Nema 8 901 (Autodesk Fusion 360 design; units mm, degrees)
Autodesk Fusion 360 part; units mm, degrees
sketch "Sketch1" plane through (0, 0, 0) normal (0, 0, 1) x (1, 0, 0)
  line L0 (10.15, -10.15) -> (-10.15, -10.15)
  line L1 (-10.15, -10.15) -> (-10.15, 10.15)
  line L2 (-10.15, 10.15) -> (10.15, 10.15)
  line L3 (10.15, 10.15) -> (10.15, -10.15)
  line L4 (10.15, -10.15) -> (-10.15, 10.15) construction
  line L5 (-10.15, -10.15) -> (10.15, 10.15) construction
  dimension "d1" = 20.3
  dimension "d2" = 20.3
  constraint perpendicular L0 L1
  constraint parallel L0 L2
  constraint parallel L1 L3
  constraint horizontal L0
  constraint coincident L4 origin
  constraint coincident L5 origin
  measures "d1" distance of L1.end L2.end
  measures "d2" distance of L0.end L1.end
extrude "Extrude1" add sketch "Sketch1" along normal blind 28
sketch "Sketch2" plane through (0, 0, 28) normal (0, 0, 1) x (-1, 0, 0)
  line L0 (-10.15, -10.15) -> (10.15, -10.15)
  line L1 (10.15, -10.15) -> (10.15, 10.15)
  line L2 (10.15, 10.15) -> (-10.15, 10.15)
  line L3 (-10.15, 10.15) -> (-10.15, -10.15)
  line L4 (-11, 11) -> (11, 11)
  line L5 (11, 11) -> (11, -11)
  line L6 (11, -11) -> (-11, -11)
  line L7 (-11, -11) -> (-11, 11)
  line L8 (-11, 11) -> (11, -11) construction
  line L9 (11, 11) -> (-11, -11) construction
  dimension "d5" = 22
  dimension "d6" = 22
  constraint perpendicular L4 L5
  constraint parallel L4 L6
  constraint parallel L5 L7
  constraint horizontal L4
  constraint coincident L8 origin
  constraint coincident L9 origin
  measures "d5" distance of L4.end L5.end
  measures "d6" distance of L5.end L6.end
extrude "Extrude2" add sketch "Sketch2" along normal blind 3 contours L0 L1 L2 L3 | L4 L5 L6 L7
sketch "Sketch3" plane through (0, 0, 31) normal (0, 0, 1) x (-1, 0, 0)
  line L0 (-11, -11) -> (11, -11)
  line L1 (11, -11) -> (11, 11)
  line L2 (11, 11) -> (-11, 11)
  line L3 (-11, 11) -> (-11, -11)
  circle A0 centre (0, 0) radius 11
  dimension "d9" = 22
  constraint coincident A0.centre origin
  measures "d9" diameter of A0
extrude "Extrude3" add sketch "Sketch3" along normal blind 24.95 contours A0
fillet "Fillet1" radius 0.5 1 faces at (0, 11, 47.6333)
sketch "Sketch4" plane through (0, 0, 55.95) normal (0, 0, 1) x (-1, 0, 0)
  circle A0 centre (0, 0) radius 11
  circle A1 centre (0, 0) radius 10.5
  constraint coincident A0.centre A1.centre
extrude "Extrude4" add sketch "Sketch4" along normal blind 3 contours A0 | A1
fillet "Fillet2" radius 0.5 1 faces at (-10.9863, 0.5483, 57.95)
fillet "Fillet3" radius 2 4 edges at (-10.15, -10.15, 14) (10.15, -10.15, 14) (10.15, 10.15, 14) (-10.15, 10.15, 14)
sketch "Sketch5" plane through (0, 0, 58.95) normal (0, 0, 1) x (-1, 0, 0)
  circle A0 centre (0, 0) radius 10.5
  circle A1 centre (0, 0) radius 6.5
  dimension "d17" = 13
  constraint coincident A0.centre A1.centre
  measures "d17" diameter of A1
extrude "Extrude5" add sketch "Sketch5" along normal blind 2 contours A1
fillet "Fillet4" radius 0.5 1 edges at (6.0601, 2.3505, 60.95)
sketch "Sketch6" plane through (0, 0, 60.95) normal (0, 0, 1) x (-1, 0, 0)
  circle A0 centre (0, 0) radius 6
  circle A1 centre (0, 0) radius 3
  dimension "d21" = 6
  constraint coincident A0.centre A1.centre
  measures "d21" diameter of A1
extrude "Extrude6" add sketch "Sketch6" along normal blind 13 contours A1
sketch "Sketch7" plane through (0, 0, 73.95) normal (0, 0, 1) x (-1, 0, 0)
  circle A0 centre (0, 0) radius 3
  line L0 (2.2361, -2) -> (-2.2361, -2)
  line L1 (0, -2) -> (0, 3) construction
  dimension "d24" = 5
  constraint coincident A0 L0.start
  constraint coincident A0 L0.end
  constraint horizontal L0
  constraint midpoint L0 L1.start
  constraint coincident A0 L1.end
  constraint perpendicular L0 L1
  measures "d24" distance of L1.start L1.end
fillet "Fillet5" radius 0.5 1 edges at (2.797, 1.0848, 73.95)
extrude "Extrude7" cut sketch "Sketch7" against normal blind 9 contours A0 L0 picked at (-0.6449, -2.0976)
sketch "Sketch9" plane through (0, 0, 0) normal (0, 0, -1) x (1, 0, 0)
  arc A0 (-10.15, -8.15) -> (-8.15, -10.15) centre (-8.15, -8.15) ccw
  line L0 (-8.15, -10.15) -> (8.15, -10.15)
  arc A1 (8.15, -10.15) -> (10.15, -8.15) centre (8.15, -8.15) ccw
  line L1 (10.15, -8.15) -> (10.15, 8.15)
  arc A2 (10.15, 8.15) -> (8.15, 10.15) centre (8.15, 8.15) ccw
  line L2 (8.15, 10.15) -> (-8.15, 10.15)
  arc A3 (-8.15, 10.15) -> (-10.15, 8.15) centre (-8.15, 8.15) ccw
  line L3 (-10.15, 8.15) -> (-10.15, -8.15)
  line L4 (-10.15, 5.15) -> (-6.65, 5.15)
  line L5 (-5.15, 6.65) -> (-5.15, 10.15)
  line L6 (-5.15, 10.15) -> (-10.15, 10.15)
  line L7 (-10.15, 10.15) -> (-10.15, 5.15)
  arc A4 (-6.65, 5.15) -> (-5.15, 6.65) centre (-6.65, 6.65) ccw
  line L8 (-5.15, -10.15) -> (-5.15, -6.65)
  arc A5 (-5.15, -6.65) -> (-6.65, -5.15) centre (-6.65, -6.65) ccw
  line L9 (-6.65, -5.15) -> (-10.15, -5.15)
  line L10 (-10.15, -5.15) -> (-10.15, -10.15)
  line L11 (-10.15, -10.15) -> (-5.15, -10.15)
  line L12 (10.15, -5.15) -> (6.65, -5.15)
  arc A6 (6.65, -5.15) -> (5.15, -6.65) centre (6.65, -6.65) ccw
  line L13 (5.15, -6.65) -> (5.15, -10.15)
  line L14 (5.15, -10.15) -> (10.15, -10.15)
  line L15 (10.15, -10.15) -> (10.15, -5.15)
  line L16 (5.15, 10.15) -> (5.15, 6.65)
  arc A7 (5.15, 6.65) -> (6.65, 5.15) centre (6.65, 6.65) ccw
  line L17 (6.65, 5.15) -> (10.15, 5.15)
  line L18 (10.15, 5.15) -> (10.15, 10.15)
  line L19 (10.15, 10.15) -> (5.15, 10.15)
  line L20 (-5.15, 10.15) -> (-10.15, 5.15) construction
  dimension "d28" = 5
  dimension "d29" = 5
  dimension "d30" = 1.5
  dimension "d32" = 360
  constraint horizontal L4
  constraint vertical L5
  constraint horizontal L6
  constraint vertical L7
  constraint coincident L2 L5.end
  constraint coincident L3 L4.start
  constraint tangent L5 A4
  constraint tangent L4 A4
  measures "d28" distance of L4.start L6.end
  measures "d29" distance of L5.end L6.end
  measures "d30" radius of A4
extrude "Extrude8" cut sketch "Sketch9" against normal blind 1.5 contours A0 L0 L3 L8 A5 L9 L10 L11 | L2 A3 L3 L4 L5 L6 L7 A4 | L0 A1 L1 L12 A6 L13 L14 L15 | L1 A2 L2 L16 A7 L17 L18 L19
chamfer "Chamfer1" distance 1.5 angle 45 4 edges at (11, -11, 29.5) (-11, -11, 29.5) (11, 11, 29.5) (-11, 11, 29.5)
